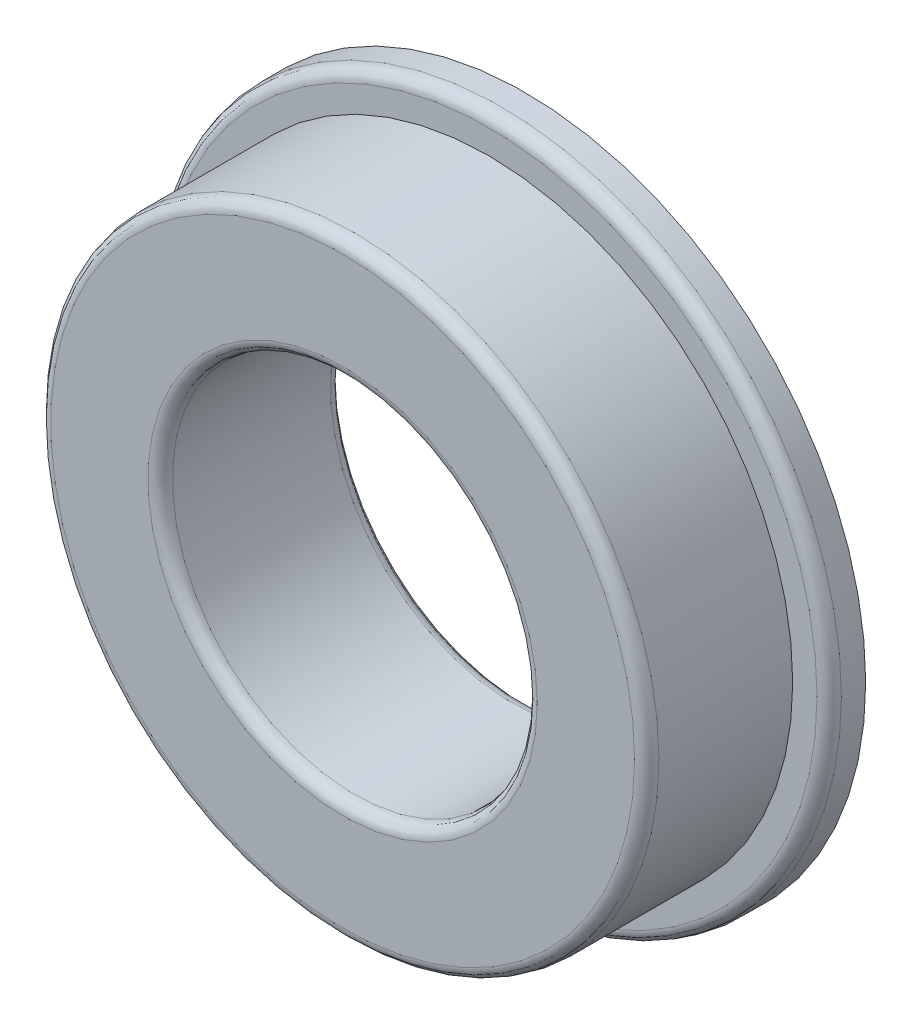
# Autodesk Inventor part: flange_bearing
Saved by Autodesk Inventor 2026.2 (Build 302298000, 298)
## iProperties
Created: 2026-03-25
Part Number: flange_bearing
Material: Generic
Document SubType Name: Modeling
Designer: szymo
Density: 1 g/cm^3
Appearance: Default
Author: szymo
Autodesk Inventor part; units mm, degrees
ref_plane "YZ Plane" through (0, 0, 0) normal (1, 0, 0) x (0, 1, 0)
ref_plane "XZ Plane" through (0, 0, 0) normal (0, 1, 0) x (-1, 0, 0)
ref_plane "XY Plane" through (0, 0, 0) normal (0, 0, 1) x (1, 0, 0)
sketch "Sketch1" plane through (0, 0, 0) normal (0, 0, 1) x (1, 0, 0)
  circle A0 centre (0, 0) radius 3
  circle A1 centre (0, 0) radius 5
  circle A2 centre (0, 0) radius 5.6
  dimension "d0" = 6
  dimension "d1" = 10
  dimension "d2" = 11.2
  constraints: 3 centre point, 3 coincident
  measures "d0" diameter of A0
  measures "d1" diameter of A1
  measures "d2" diameter of A2
extrude "Extrusion1" add sketch "Sketch1" along normal blind 3 contours A1
extrude "Extrusion2" add sketch "Sketch1" along normal blind 0.6 contours A2
fillet "Fillet1" radius 0.2 4 edges at (-5.6, 0, 0.6) (-5, 0, 3) (-3, 0, 3) (-3, 0, 0)
body "Solid1"
